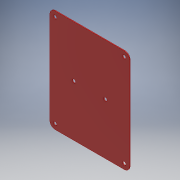
# Autodesk Inventor part: SolarPanel_PCB
Saved by Autodesk Inventor 2017 (Build 210142000, 142)
## iProperties
Created: 2018-05-13
Part Number: SolarPanel_PCB
Material: Fiberglass Batt
Document SubType Name: Modeling
Designer: Bradley
Density: 0.032 g/cm^3
Appearance: Smooth - Red
Author: Bradley
Autodesk Inventor part; units mm, degrees
ref_plane "YZ Plane" through (0, 0, 0) normal (1, 0, 0) x (0, 1, 0)
ref_plane "XZ Plane" through (0, 0, 0) normal (0, 1, 0) x (-1, 0, 0)
ref_plane "XY Plane" through (0, 0, 0) normal (0, 0, 1) x (1, 0, 0)
sketch "Sketch1" plane through (0, 0, 0) normal (0, 1, 0) x (-1, 0, 0)
  line L0 (50, 57) -> (41.5, 57) construction
  line L1 (41.5, 57) -> (41.5, -56.5) construction
  line L2 (41.5, -56.5) -> (50, -56.5) construction
  line L3 (50, -56.5) -> (50, 57) construction
  line L4 (-41.5, 57) -> (-50, 57) construction
  line L5 (-50, 57) -> (-50, -56.5) construction
  line L6 (-50, -56.5) -> (-41.5, -56.5) construction
  line L7 (-41.5, -56.5) -> (-41.5, 57) construction
  line L8 (41.5, 50) -> (-41.5, 50) construction
  line L9 (-41.5, 50) -> (-41.5, -50) construction
  line L10 (-41.5, -50) -> (41.5, -50) construction
  line L11 (41.5, -50) -> (41.5, 50) construction
  line L12 (0, 50) -> (0, -50) construction
  line L13 (33, 49) -> (-33, 49)
  line L14 (-38, 44) -> (-38, -44)
  line L15 (-33, -49) -> (33, -49)
  line L16 (38, -44) -> (38, 44)
  line L17 (34.5, 5) -> (-34.5, 5) construction
  line L18 (-34.5, 5) -> (-34.5, 36.7) construction
  line L19 (-34.5, 36.7) -> (-26.5, 44.7) construction
  line L20 (-26.5, 44.7) -> (26.5, 44.7) construction
  line L21 (26.5, 44.7) -> (34.5, 36.7) construction
  line L22 (34.5, 36.7) -> (34.5, 5) construction
  line L23 (34.5, -5) -> (-34.5, -5) construction
  line L24 (-34.5, -5) -> (-34.5, -36.7) construction
  line L25 (-34.5, -36.7) -> (-26.5, -44.7) construction
  line L26 (-26.5, -44.7) -> (26.5, -44.7) construction
  line L27 (26.5, -44.7) -> (34.5, -36.7) construction
  line L28 (34.5, -36.7) -> (34.5, -5) construction
  line L29 (0, 5) -> (0, -5) construction
  circle A0 centre (33, 44) radius 2.85 construction
  circle A1 centre (33, 44) radius 1.65
  circle A2 centre (33, 44) radius 1.5 construction
  line L30 (33, 44) -> (-33, 44) construction
  line L31 (-33, 44) -> (-33, -44) construction
  line L32 (-33, -44) -> (33, -44) construction
  line L33 (33, -44) -> (33, 44) construction
  circle A3 centre (-33, -44) radius 1.65
  circle A4 centre (33, -44) radius 1.65
  circle A5 centre (-33, 44) radius 1.65
  line L34 (15, 0) -> (-15, 0) construction
  circle A6 centre (15, 0) radius 1.65
  circle A7 centre (-15, 0) radius 1.65
  arc A8 (38, 44) -> (33, 49) centre (33, 44) ccw
  arc A9 (-33, 49) -> (-38, 44) centre (-33, 44) ccw
  arc A10 (-38, -44) -> (-33, -49) centre (-33, -44) ccw
  arc A11 (33, -49) -> (38, -44) centre (33, -44) ccw
  point P0 (0, 0)
  point P1 (0, 0)
  point P2 (38, 49)
  point P3 (-38, -49)
  point P4 (-38, 49)
  point P5 (38, -49)
  point P6 (0, 49)
  point P7 (0, 44.7)
  point P8 (38, 0)
  point P9 (0, 44)
  point P10 (33, 0)
  dimension "d0" = 100
  dimension "d1" = 8.5
  dimension "d2" = 100
  dimension "d3" = 6.5
  dimension "d4" = 7
  dimension "d5" = 12
  dimension "d6" = 10
  dimension "d7" = 69
  dimension "d8" = 39.7
  dimension "d10" = 8
  dimension "d11" = 3
  dimension "d12" = 3.3
  dimension "d13" = 5.7
  dimension "d14" = 30
  dimension "d17" = 98
  dimension "d18" = 76
  dimension "d19" = 66
  dimension "d20" = 88
  dimension "d21" = 1.2512
  dimension "d22" = 5
  constraints: 70 end point, 16 point on line, 15 parallel, 12 centre point, 12 midpoint, 9 perpendicular, 8 coincident, 8 equal radius, 8 point on circle, 8 tangent, 7 horizontal, 6 equal length, 3 vertical alignment, 2 horizontal alignment
  measures "d0" distance between parallel lines of L5 L3
  measures "d1" distance of L0.start L0.end
  measures "d2" distance between parallel lines of L10 L8
  measures "d3" distance between parallel lines of L2 L10
  measures "d4" distance between parallel lines of L8 L0
  measures "d5" distance between parallel lines of L16 L3
  measures "d6" distance between parallel lines of L23 L17
  measures "d7" distance of L17.start L17.end
  measures "d8" distance between parallel lines of L17 L20
  measures "d10" horizontal distance of L18.end L19.end
  measures "d11" diameter of A2
  measures "d12" diameter of A1
  measures "d13" diameter of A0
  measures "d14" distance of L34.start L34.end
  measures "d17" distance of point (38, -49) point (38, 49)
  measures "d18" distance of point (38, 49) point (-38, 49)
  measures "d19" distance of L30.start L30.end
  measures "d20" distance of L32.end L30.start
  measures "d21" distance edge to line of A0 L21
  measures "d22" radius of A8
extrude "Extrusion1" add sketch "Sketch1" along normal mid plane 0.6
body "Solid1"
